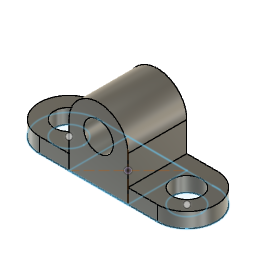
A4 (Autodesk Fusion 360 design; units mm, degrees)
Autodesk Fusion 360 part; units mm, degrees
sketch "Sketch2" plane through (0, 0, 0) normal (0, 0, 1) x (1, 0, 0)
  circle A0 centre (-40, 0) radius 10
  circle A1 centre (40, 0) radius 10
  line L0 (-40, 20) -> (42.4572, 19.8485)
  line L1 (-40, -20) -> (40, -20)
  line L2 (20, -20) -> (-20, -20)
  line L3 (-20, -20) -> (-20, 20)
  line L4 (-20, 20) -> (20, 20)
  line L5 (20, 20) -> (20, -20)
  line L6 (20, -20) -> (-20, 20) construction
  line L7 (-20, -20) -> (20, 20) construction
  arc A2 (-39.9265, 19.9999) -> (-40, -20) centre (-40, 0) ccw
  arc A3 (40, -20) -> (37.6158, 19.8574) centre (40, 0) ccw
  dimension "d3" = 20
  dimension "d4" = 20
  dimension "d7" = 40
  dimension "d8" = 40
  constraint coincident L0.start A2
  constraint coincident L0.end A3
  constraint tangent L1 A2
  constraint horizontal L1
  constraint horizontal L2
  constraint perpendicular L2 L3
  constraint parallel L2 L4
  constraint parallel L3 L5
  constraint coincident L6 origin
  constraint coincident L7 origin
  constraint concentric A0 A2
  constraint coincident L0 A2.start
  constraint concentric A1 A3
  constraint coincident L0 A3.end
  measures "d3" diameter of A0
  measures "d4" diameter of A1
  measures "d7" distance of L3.end L4.end
  measures "d8" distance of L2.end L3.end
extrude "Extrude2" add sketch "Sketch2" along normal blind 50 contours L0 L1 L2 L3 L5 makes body 1
extrude "Extrude1" add sketch "Sketch2" along normal blind 10 separate body contours L0 L1 L3 A2 | L0 L1 L5 A3 makes body 2 at (-23.3333, -0.0122, 0) makes body 3 at (23.3333, -0.0367, 0)
sketch "Sketch3" plane through (0, -20, 0) normal (0, -1, 0) x (1, 0, 0)
  line L0 (-20, 0) -> (20, 0)
  line L1 (20, 0) -> (20, 50)
  line L2 (20, 50) -> (-20, 50)
  line L3 (-20, 50) -> (-20, 0)
  circle A0 centre (0, 30) radius 10
  arc A1 (20, 30) -> (-20, 30) centre (0, 30) ccw
  dimension "d13" = 20
  constraint concentric A0 A1
  constraint coincident L3 A1.end
  constraint coincident L1 A1.start
  measures "d13" diameter of A0
extrude "Extrude5" cut sketch "Sketch3" against normal blind 40 contours A0 bodies 1
extrude "Extrude4" cut sketch "Sketch3" against normal blind 40 contours L1 L2 A1 bodies 1
extrude "Extrude3" cut sketch "Sketch3" against normal blind 40 contours L2 L3 A1 bodies 1
